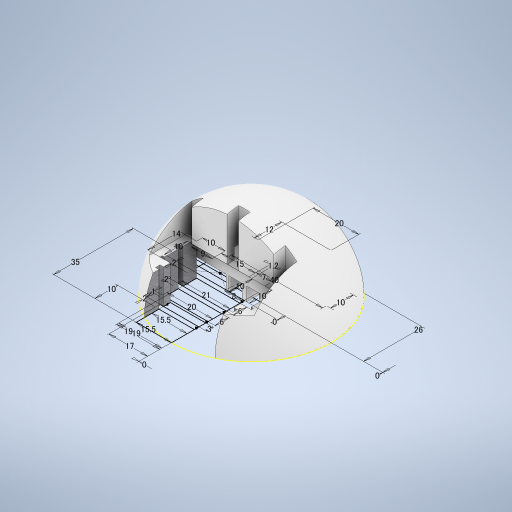
# Autodesk Inventor part: body back for tire1
Saved by Autodesk Inventor 2023 (Build 270158000, 158)
## iProperties
Created: 2022-10-08
Part Number: body back for tire1
Material: ABS プラスチック
Document SubType Name: Modeling
Designer: ellie
Density: 1.06 g/cm^3
Appearance: 積雪
Author: ellie
Autodesk Inventor part; units mm, degrees
sketch "スケッチ1" plane through (0, 0, 0) normal (0, 1, 0) x (-1, 0, 0)
  circle A0 centre (0, 0) radius 35
  line L0 (0, 0) -> (0, -35)
  line L1 (0, 0) -> (0, 35)
  dimension "d0" = 70
  constraints: 4 end point, 2 point on circle, 2 vertical, 1 centre point, 1 coincident
  measures "d0" diameter of A0
revolve "回転1" add sketch "スケッチ1" angle 180 about axis through (0, 0, 0) along (0, 0, 1) picked at (-2.5961, -23.0408) contours L1 L0 A0
sketch "スケッチ5" plane through (0, 0, 0) normal (0, -1, 0) x (1, 0, 0)
  line L0 (-20, -23) -> (20, -23)
  line L1 (20, -23) -> (20, -13)
  line L2 (20, -13) -> (-20, -13)
  line L3 (-20, -13) -> (-20, -23)
  line L4 (-20, -15) -> (-20, -13)
  line L5 (0, 25) -> (-17, 25)
  line L6 (-17, 25) -> (-17, 23)
  line L7 (-17, 23) -> (0, 23)
  line L8 (0, 23) -> (0, 25)
  line L9 (0, 20) -> (-20, 20)
  line L10 (-20, 20) -> (-20, 19)
  line L11 (-20, 19) -> (0, 19)
  line L12 (0, 19) -> (0, 20)
  line L13 (0, 13) -> (-21, 13)
  line L14 (-21, 13) -> (-21, 11)
  line L15 (-21, 11) -> (0, 11)
  line L16 (0, 11) -> (0, 13)
  line L17 (0, 5) -> (-23, 5)
  line L18 (-23, 5) -> (-23, 3)
  line L19 (-23, 3) -> (0, 3)
  line L20 (0, 3) -> (0, 5)
  circle A0 centre (0, 0) radius 35 projected
  circle A1 centre (0, 0) radius 35 projected
  line L21 (0, 35) -> (0, -35)
  line L22 (35, 0) -> (-35, 0)
  line L23 (-32, 3) -> (-23, 3)
  line L24 (-23, 3) -> (-23, -7)
  line L25 (-23, -7) -> (-32, -7)
  line L26 (-32, -7) -> (-32, 3)
  line L27 (-23, -8.0262) -> (-23, 3)
  line L28 (-15.5, 25) -> (0, 25)
  line L29 (0, 25) -> (0, 35)
  line L30 (0, 35) -> (-15.5, 35)
  line L31 (-15.5, 35) -> (-15.5, 25)
  line L32 (-15.5, 23) -> (0, 23)
  line L33 (0, 23) -> (0, 20)
  line L34 (0, 20) -> (-15.5, 20)
  line L35 (-15.5, 20) -> (-15.5, 23)
  line L36 (-19, 13) -> (0, 13)
  line L37 (0, 13) -> (0, 19)
  line L38 (0, 19) -> (-19, 19)
  line L39 (-19, 19) -> (-19, 13)
  line L40 (-19, 11) -> (0, 11)
  line L41 (0, 11) -> (0, 5)
  line L42 (0, 5) -> (-19, 5)
  line L43 (-19, 5) -> (-19, 11)
  line L44 (-23, -2) -> (-39.6865, -2)
  line L45 (-23, -2) -> (-7.8337, -2)
  line L46 (-8, 3) -> (-23, 3)
  line L47 (-23, 3) -> (-23, -7)
  line L48 (-23, -7) -> (-8, -7)
  line L49 (-8, -7) -> (-8, 3)
  line L50 (-8, 3) -> (-23, -7) construction
  line L51 (-23, 3) -> (-8, -7) construction
  line L52 (-23, 5) -> (-33, 5)
  line L53 (-33, 5) -> (-33, -9)
  line L54 (-33, -9) -> (-23, -9)
  line L55 (-23, -9) -> (-23, 5)
  line L56 (-23, 5) -> (-33, -9) construction
  line L57 (-33, 5) -> (-23, -9) construction
  line L58 (-8, 3) -> (-1, 3)
  line L59 (-1, 3) -> (-1, -7)
  line L60 (-1, -7) -> (-8, -7)
  line L61 (-8, -7) -> (-8, 3)
  line L62 (-8, 3) -> (-1, -7) construction
  line L63 (-1, 3) -> (-8, -7) construction
  line L64 (-23, 3) -> (-27, 3)
  line L65 (-23, -7) -> (-27, -7)
  line L66 (-23, 5) -> (-27, 5)
  line L67 (-23, -9) -> (-27, -9)
  line L68 (23.4307, -26) -> (-23.4307, -26)
  line L69 (-8, 3) -> (-6.8, 3)
  line L70 (-6.8, 3) -> (-6.8, -7)
  line L71 (-6.8, -7) -> (-8, -7)
  line L72 (-8, -7) -> (-8, 3)
  line L73 (-3, 5) -> (0, 5)
  line L74 (0, 20) -> (-4, 20)
  line L75 (-4, 19) -> (0, 19)
  line L76 (0, 19) -> (0, 20)
  line L77 (-6, 5) -> (-1, 5)
  line L78 (-1, 3) -> (-6, 3)
  line L79 (-33, -11.6619) -> (-33, 11.6619)
  point P0 (0, -23)
  point P1 (0, -13)
  point P2 (0, 24)
  point P3 (0, 19.5)
  point P4 (0, 12)
  point P5 (0, 4)
  point P6 (-20, -18)
  point P7 (-15.5, 21.5)
  point P8 (-15.5, 31.3807)
  point P9 (0, 25)
  point P10 (0, 23)
  point P11 (0, 11)
  point P12 (0, 13)
  point P13 (-32, 0)
  point P14 (-23, 0)
  point P15 (-15.5, -2)
  point P16 (-28, -2)
  point P17 (-4.5, -2)
  point P18 (-8, 3)
  point P19 (-28, 0.4738)
  point P20 (-28, -11.5262)
  point P21 (-23, -7)
  point P22 (-23, -7)
  point P23 (-23, -7)
  point P24 (-8, 0)
  point P25 (-1, 0)
  point P26 (0, 19)
  point P27 (0, 20)
  point P28 (-34.9428, -2)
  point P29 (-33, 11.6619)
  dimension "d12" = 40
  dimension "d13" = 10
  dimension "d23" = 17
  dimension "d24" = 2
  dimension "d27" = 20
  dimension "d28" = 1
  dimension "d30" = 21
  dimension "d31" = 2
  dimension "d33" = 2
  dimension "d88" = 0
  dimension "d89" = 0
  dimension "d90" = 12
  dimension "d92" = 20
  dimension "d93" = 10
  dimension "d97" = 9
  dimension "d98" = 10
  dimension "d122" = 15.5
  dimension "d123" = 35
  dimension "d124" = 3
  dimension "d125" = 15.5
  dimension "d126" = 6
  dimension "d127" = 6
  dimension "d128" = 19
  dimension "d129" = 19
  dimension "d147" = 10
  dimension "d149" = 8
  dimension "d151" = 15
  dimension "d161" = 14
  dimension "d162" = 10
  dimension "d164" = 10
  dimension "d165" = 7
  dimension "d170" = 26
  dimension "d175" = 1.2
  dimension "d207" = 0
  constraints: 158 end point, 31 parallel, 20 horizontal, 15 midpoint, 15 point on line, 14 perpendicular, 10 collinear, 21 other
  measures "d12" distance of L2.end L1.end
  measures "d13" distance of L1.end L0.end
  measures "d23" distance of L7.end L6.end
  measures "d24" distance of L6.end L5.end
  measures "d27" distance of L11.end L10.end
  measures "d28" distance of L10.end L9.end
  measures "d30" distance of L15.end L14.end
  measures "d31" distance of L14.end L13.end
  measures "d33" distance of L18.end L17.end
  measures "d89" distance from line of point (0, 0) L22
  measures "d90" distance from line of L0 point (0, -35)
  measures "d92" distance of the line from the sketch origin of L3
  measures "d93" distance from line of L5 point (0, 35)
  measures "d97" distance of L24.end L25.end
  measures "d98" distance of L23.end L24.end
  measures "d122" distance of the line from the sketch origin of L31
  measures "d123" distance between parallel lines of L30 L22
  measures "d124" distance of L32.end L33.end
  measures "d126" distance of L37.end L36.end
  measures "d127" distance of L40.end L41.end
  measures "d128" distance of the line from the sketch origin of L43
  measures "d129" distance of the line from the sketch origin of L39
  measures "d147" distance of L47.end L46.end
  measures "d149" distance of the line from the sketch origin of L49
  measures "d151" distance between parallel lines of L49 L24
  measures "d161" distance between parallel lines of L54 L52
  measures "d162" distance between parallel lines of L47 L53
  measures "d164" distance between parallel lines of L60 L58
  measures "d165" distance between parallel lines of L49 L59
  measures "d170" distance between parallel lines of L68 L22
  measures "d175" distance of L70.end L71.end
  measures "d207" distance between parallel lines of L46 L19
extrude "GNSボード" cut sketch "スケッチ5" against normal blind 16 contours L8 L7 L6 L5
extrude "GNSボード止めるよう" cut sketch "スケッチ5" against normal blind 15 contours L21 L5 L31 A0 | L21 L9 L35 L7
extrude "アルミ板１" cut sketch "スケッチ5" against normal blind 20 contours L11 L10 L9 L12
extrude "メイン基板" cut sketch "スケッチ5" against normal blind 21 contours L15 L14 L13 L16
extrude "メイン止めるよう" cut sketch "スケッチ5" against normal blind 15 contours L17 L43 L15 L21 | L13 L39 L11 L21
extrude "アルミ板２" cut sketch "スケッチ5" against normal blind 20 contours L19 L18 L17 L20
extrude "電池ボックス入れ" cut sketch "スケッチ5" against normal blind 13 contours L3 L2 L21 L0 | L21 L2 L1 L0
extrude "motor case" add sketch "スケッチ5" against normal blind 7 contours L53 L44 L26 L25 L27 L55 L54 | L49 L45 L24 L22 | L22 L24 L19 L49 | L53 L22 L26 L44 | L24 L44 L26 L22 | L22 L26 L23 L24 | L49 L48 L24 L45 | L53 L52 L18 L23 L26 L22 | L44 L24 L25 L26
extrude "bottom cut" cut sketch "スケッチ5" against normal blind 90 contours L68 A0 L21 | L21 A0 L68
extrude "motor" cut sketch "スケッチ5" against normal blind 6 contours L59 L60 L70 L22 | L22 L70 L19 L59 | L70 L60 L49 L22 | L22 L49 L19 L70 | L49 L45 L24 L22 | L22 L24 L19 L49 | L24 L44 L26 L22 | L22 L26 L23 L24 | L49 L48 L24 L45 | L44 L24 L25 L26
extrude "motor block" add sketch "スケッチ5" against normal blind 10 contours L70 L60 L49 L22 | L22 L49 L19 L70
mirror "ミラー13" about plane through (0, 0, 0) normal (1, 0, 0) of "メイン止めるよう", "メイン基板", "アルミ板１", "GNSボード止めるよう", "GNSボード", "アルミ板２", "motor", "motor case", "電池ボックス入れ", "motor block"
ref_plane "作業平面5" through (-17, 17.5, 23) normal (0, -1, 0) x (1, 0, 0)
ref_plane "作業平面6" through (20, 13, -13) normal (0, 0, -1) x (1, 0, 0)
ref_plane "作業平面7" through (27, 35, 5) normal (0, -1, 0) x (1, 0, 0)
sketch "スケッチ41" plane through (-17, 0, 23) normal (0, -1, 0) x (1, 0, 0)
  line L0 (-15, -30) -> (-15, -20) projected
  line L1 (-15, -20) -> (-6, -20) projected
  line L2 (-6, -20) -> (-6, -18) projected
  line L3 (-6, -18) -> (-2, -18) projected
  line L4 (-2, -18) -> (-2, -12) projected
  line L5 (-2, -12) -> (-4, -12) projected
  line L6 (-4, -12) -> (-4, -10) projected
  line L7 (-4, -10) -> (-2, -10) projected
  line L8 (-2, -10) -> (-2, -4) projected
  line L9 (-2, -4) -> (-3, -4) projected
  line L10 (-3, -4) -> (-3, -3) projected
  line L11 (-3, -3) -> (1.5, -3) projected
  line L12 (1.5, -3) -> (1.5, 0) projected
  line L13 (1.5, 0) -> (0, 0) projected
  line L14 (0, 0) -> (0, 2) projected
  line L15 (0, 2) -> (1.5, 2) projected
  line L16 (1.5, 2) -> (1.5, 8.3807) projected
  arc A0 (1.5, 8.3807) -> (-6.4307, -49) centre (17, -23) ccw projected
  line L17 (-2, -18) -> (-2, -12) projected
  line L18 (-4, -10) -> (-4, -12) projected
  line L19 (0, 2) -> (0, 0) projected
  circle A1 centre (-4, 0.5) radius 2.4
  line L20 (18, -30) -> (18, -20) projected
  line L21 (18, -20) -> (16, -20) projected
  line L22 (16, -20) -> (16, -30) projected
  line L23 (16, -30) -> (10.2, -30) projected
  line L24 (10.2, -30) -> (10.2, -20) projected
  line L25 (10.2, -20) -> (9, -20) projected
  line L26 (9, -20) -> (9, -30) projected
  line L27 (9, -30) -> (-15, -30) projected
  line L28 (-6.4307, -49) -> (40.4307, -49) projected
  arc A2 (40.4307, -49) -> (32.5, 8.3807) centre (17, -23) ccw projected
  line L29 (32.5, 8.3807) -> (32.5, 2) projected
  line L30 (32.5, 2) -> (34, 2) projected
  line L31 (34, 2) -> (34, 0) projected
  line L32 (34, 0) -> (32.5, 0) projected
  line L33 (32.5, 0) -> (32.5, -3) projected
  line L34 (32.5, -3) -> (37, -3) projected
  line L35 (37, -3) -> (37, -4) projected
  line L36 (37, -4) -> (36, -4) projected
  line L37 (36, -4) -> (36, -10) projected
  line L38 (36, -10) -> (38, -10) projected
  line L39 (38, -10) -> (38, -12) projected
  line L40 (38, -12) -> (36, -12) projected
  line L41 (36, -12) -> (36, -18) projected
  line L42 (36, -18) -> (40, -18) projected
  line L43 (40, -18) -> (40, -20) projected
  line L44 (40, -20) -> (49, -20) projected
  line L45 (49, -20) -> (49, -30) projected
  line L46 (49, -30) -> (25, -30) projected
  line L47 (25, -20) -> (25, -30) projected
  line L48 (23.8, -20) -> (25, -20) projected
  line L49 (23.8, -30) -> (23.8, -20) projected
  line L50 (23.8, -30) -> (18, -30) projected
  dimension "d252" = 4.8
  dimension "d253" = 4
  dimension "d254" = 3.5
  constraints: 1 centre point
  measures "d252" diameter of A1
  measures "d253" distance from line of A1.centre L14
  measures "d254" distance from line of A1.centre L11
extrude "top lock 10mm" cut sketch "スケッチ41" against normal blind 3 contours A1
mirror "ミラー15" about plane through (0, 0, 0) normal (1, 0, 0) of "top lock 10mm"
ref_plane "作業平面9" through (-33, 0, -9) normal (0, -1, 0) x (1, 0, 0)
sketch "スケッチ42" plane through (-33, 0, -9) normal (0, -1, 0) x (1, 0, 0)
  circle A0 centre (9.5, -3) radius 2.4
  line L0 (13, -14) -> (13, -4) projected
  line L1 (32, 2) -> (1, 2) projected
  point P0 (33, 9)
  point P1 (10, 2)
  dimension "d257" = 3.5
  dimension "d258" = 4.8
  dimension "d259" = 5
  constraints: 1 centre point
  measures "d257" distance from line of A0.centre L0
  measures "d258" diameter of A0
  measures "d259" distance from line of A0.centre L1
extrude "bottom lock" cut sketch "スケッチ42" against normal blind 3
ref_plane "作業平面8" through (-17, 15, 23) normal (0, -1, 0) x (1, 0, 0)
sketch "スケッチ45" plane through (-17, 15, 23) normal (0, -1, 0) x (1, 0, 0)
  circle A0 centre (-4, 0.5) radius 2.4 projected
  line L0 (-15, -30) -> (-15, -20) projected
  line L1 (-15, -20) -> (-6, -20) projected
  line L2 (-6, -20) -> (-6, -18) projected
  line L3 (-6, -18) -> (-2, -18) projected
  line L4 (-2, -18) -> (-2, -12) projected
  line L5 (-2, -12) -> (-4, -12) projected
  line L6 (-4, -12) -> (-4, -10) projected
  line L7 (-4, -10) -> (-2, -10) projected
  line L8 (-2, -10) -> (-2, -4) projected
  line L9 (-2, -4) -> (-3, -4) projected
  line L10 (-3, -4) -> (-3, -3) projected
  line L11 (-3, -3) -> (1.5, -3) projected
  line L12 (1.5, -3) -> (1.5, 0) projected
  line L13 (1.5, 0) -> (0, 0) projected
  line L14 (0, 0) -> (0, 2) projected
  line L15 (0, 2) -> (1.5, 2) projected
  line L16 (1.5, 2) -> (1.5, 8.3807) projected
  arc A1 (1.5, 8.3807) -> (-6.4307, -49) centre (17, -23) ccw projected
  arc A2 (32.5, 4.5636) -> (1.5, 4.5636) centre (17, -23) ccw projected
  line L17 (1.5, 2) -> (1.5, 4.5636) projected
  line L18 (32.5, 2) -> (1.5, 2) projected
  line L19 (32.5, 2) -> (32.5, 4.5636) projected
  circle A3 centre (38, 0.5) radius 2.4 projected
  arc A4 (40.4307, -49) -> (32.5, 8.3807) centre (17, -23) ccw projected
  line L20 (32.5, 8.3807) -> (32.5, 2) projected
  line L21 (32.5, 2) -> (34, 2) projected
  line L22 (34, 2) -> (34, 0) projected
  line L23 (34, 0) -> (32.5, 0) projected
  line L24 (32.5, 0) -> (32.5, -3) projected
  line L25 (32.5, -3) -> (37, -3) projected
  line L26 (37, -3) -> (37, -4) projected
  line L27 (37, -4) -> (36, -4) projected
  line L28 (36, -4) -> (36, -10) projected
  line L29 (36, -10) -> (38, -10) projected
  line L30 (38, -10) -> (38, -12) projected
  line L31 (38, -12) -> (36, -12) projected
  line L32 (36, -12) -> (36, -18) projected
  line L33 (36, -18) -> (40, -18) projected
  line L34 (40, -18) -> (40, -20) projected
  line L35 (40, -20) -> (49, -20) projected
  line L36 (49, -20) -> (49, -30) projected
  circle A5 centre (38, 0.5) radius 2.4 projected
  circle A6 centre (-4, 0.5) radius 2.4 projected
  line L37 (34, 0) -> (0, 0) projected
  line L38 (34, 0) -> (34, 2) projected
  line L39 (34, 2) -> (0, 2) projected
  line L40 (0, 0) -> (0, 2) projected
  line L41 (32.5, -3) -> (1.5, -3) projected
  line L42 (32.5, -3) -> (32.5, 0) projected
  line L43 (1.5, 0) -> (32.5, 0) projected
  line L44 (1.5, -3) -> (1.5, 0) projected
  line L45 (-2, -4) -> (36, -4) projected
  circle A7 centre (38, 0.5) radius 2.4 projected
  line L46 (36, -10) -> (-2, -10) projected
  line L47 (36, -10) -> (36, -4) projected
  line L48 (-2, -4) -> (36, -4) projected
  line L49 (-2, -10) -> (-2, -4) projected
  line L50 (-2, -12) -> (36, -12) projected
  line L51 (36, -18) -> (-2, -18) projected
  line L52 (36, -18) -> (36, -12) projected
  line L53 (-2, -12) -> (36, -12) projected
  line L54 (-2, -18) -> (-2, -12) projected
  line L55 (40, -20) -> (-6, -20) projected
  line L56 (40, -20) -> (40, -18) projected
  line L57 (40, -18) -> (-6, -18) projected
  line L58 (-6, -20) -> (-6, -18) projected
  line L59 (9, -30) -> (9, -20) projected
  line L60 (-6, -20) -> (9, -20) projected
  line L61 (-15, -20) -> (-6, -20) projected
  line L62 (-15, -30) -> (-15, -20) projected
  line L63 (16, -30) -> (10.2, -30) projected
  line L64 (18, -30) -> (18, -20) projected
  line L65 (18, -20) -> (16, -20) projected
  line L66 (16, -20) -> (16, -30) projected
  line L67 (-6, -20) -> (-6, -18) projected
  line L68 (16, -30) -> (10.2, -30) projected
  line L69 (-15, -30) -> (-15, -20) projected
  arc A8 (1.5, 8.3807) -> (-6.4307, -49) centre (17, -23) ccw projected
  line L70 (-6.4307, -49) -> (40.4307, -49) projected
  arc A9 (40.4307, -49) -> (32.5, 8.3807) centre (17, -23) ccw projected
  line L71 (49, -20) -> (49, -30) projected
  line L72 (23.8, -30) -> (18, -30) projected
  line L73 (40, -18) -> (40, -20) projected
  line L74 (-3, -36) -> (37, -36) projected
  line L75 (37, -36) -> (37, -46) projected
  line L76 (37, -46) -> (-3, -46) projected
  line L77 (-3, -46) -> (-3, -36) projected
  line L78 (-6, -15) -> (40, -15)
  line L79 (40, -15) -> (40, 8.6228)
  line L80 (40, 8.6228) -> (-6, 8.6228)
  line L81 (-6, 8.6228) -> (-6, -15)
  line L82 (10.2, -20) -> (10.2, -30) projected
  line L83 (16, -20) -> (16, -30) projected
  line L84 (10.2, -20) -> (16, -20) projected
  line L85 (9, -30) -> (-15, -30) projected
  line L86 (-15, -20) -> (-6, -20) projected
  line L87 (-6, -18) -> (-2, -18) projected
  line L88 (-2, -18) -> (-2, -12) projected
  line L89 (-2, -12) -> (-4, -12) projected
  line L90 (-4, -12) -> (-4, -10) projected
  line L91 (-4, -10) -> (-2, -10) projected
  line L92 (-2, -10) -> (-2, -4) projected
  line L93 (-2, -4) -> (-3, -4) projected
  line L94 (-3, -4) -> (-3, -3) projected
  line L95 (-3, -3) -> (1.5, -3) projected
  line L96 (1.5, -3) -> (1.5, 0) projected
  line L97 (1.5, 0) -> (0, 0) projected
  line L98 (0, 0) -> (0, 2) projected
  line L99 (0, 2) -> (1.5, 2) projected
  line L100 (1.5, 2) -> (1.5, 8.3807) projected
  line L101 (10.2, -30) -> (10.2, -20) projected
  line L102 (10.2, -20) -> (9, -20) projected
  line L103 (9, -20) -> (9, -30) projected
  line L104 (9, -30) -> (-15, -30) projected
  line L105 (49, -30) -> (25, -30) projected
  line L106 (25, -20) -> (25, -30) projected
  line L107 (23.8, -20) -> (25, -20) projected
  line L108 (23.8, -30) -> (23.8, -20) projected
  line L109 (32.5, 8.3807) -> (32.5, 2) projected
  line L110 (32.5, 2) -> (34, 2) projected
  line L111 (34, 2) -> (34, 0) projected
  line L112 (34, 0) -> (32.5, 0) projected
  line L113 (32.5, 0) -> (32.5, -3) projected
  line L114 (32.5, -3) -> (37, -3) projected
  line L115 (37, -3) -> (37, -4) projected
  line L116 (37, -4) -> (36, -4) projected
  line L117 (36, -4) -> (36, -10) projected
  line L118 (36, -10) -> (38, -10) projected
  line L119 (38, -10) -> (38, -12) projected
  line L120 (38, -12) -> (36, -12) projected
  line L121 (36, -12) -> (36, -18) projected
  line L122 (36, -18) -> (40, -18) projected
  line L123 (40, -20) -> (49, -20) projected
  line L124 (18, -30) -> (18, -20) projected
  line L125 (18, -20) -> (16, -20) projected
  line L126 (16, -20) -> (16, -30) projected
  line L127 (16, -30) -> (10.2, -30) projected
  line L128 (10.2, -30) -> (10.2, -20) projected
  line L129 (10.2, -20) -> (9, -20) projected
  line L130 (9, -20) -> (9, -30) projected
  line L131 (9, -30) -> (-15, -30) projected
  line L132 (-15, -30) -> (-15, -20) projected
  line L133 (-15, -20) -> (-6, -20) projected
  line L134 (-6, -20) -> (-6, -18) projected
  line L135 (-6, -18) -> (-2, -18) projected
  line L136 (-2, -18) -> (-2, -12) projected
  line L137 (-2, -12) -> (-4, -12) projected
  line L138 (-4, -12) -> (-4, -10) projected
  line L139 (-4, -10) -> (-2, -10) projected
  line L140 (-2, -10) -> (-2, -4) projected
  line L141 (-2, -4) -> (-3, -4) projected
  line L142 (-3, -4) -> (-3, -3) projected
  line L143 (-3, -3) -> (1.5, -3) projected
  line L144 (1.5, -3) -> (1.5, 0) projected
  line L145 (1.5, 0) -> (0, 0) projected
  line L146 (0, 0) -> (0, 2) projected
  line L147 (0, 2) -> (1.5, 2) projected
  line L148 (1.5, 2) -> (1.5, 8.3807) projected
  arc A10 (1.5, 8.3807) -> (-6.4307, -49) centre (17, -23) ccw projected
  line L149 (-6.4307, -49) -> (40.4307, -49) projected
  line L150 (49, -30) -> (25, -30) projected
  line L151 (25, -20) -> (25, -30) projected
  line L152 (23.8, -20) -> (25, -20) projected
  line L153 (23.8, -30) -> (23.8, -20) projected
  line L154 (23.8, -30) -> (18, -30) projected
  line L155 (18, -30) -> (18, -20) projected
  line L156 (18, -20) -> (16, -20) projected
  line L157 (16, -20) -> (16, -30) projected
  line L158 (16, -30) -> (10.2, -30) projected
  line L159 (10.2, -30) -> (10.2, -20) projected
  line L160 (10.2, -20) -> (9, -20) projected
  line L161 (9, -20) -> (9, -30) projected
  line L162 (9, -30) -> (-15, -30) projected
  line L163 (-6.4307, -49) -> (40.4307, -49) projected
  arc A11 (40.4307, -49) -> (32.5, 8.3807) centre (17, -23) ccw projected
  line L164 (32.5, 8.3807) -> (32.5, 2) projected
  line L165 (32.5, 2) -> (34, 2) projected
  line L166 (34, 2) -> (34, 0) projected
  line L167 (34, 0) -> (32.5, 0) projected
  line L168 (32.5, 0) -> (32.5, -3) projected
  line L169 (32.5, -3) -> (37, -3) projected
  line L170 (37, -3) -> (37, -4) projected
  line L171 (37, -4) -> (36, -4) projected
  line L172 (36, -4) -> (36, -10) projected
  line L173 (36, -10) -> (38, -10) projected
  line L174 (38, -10) -> (38, -12) projected
  line L175 (38, -12) -> (36, -12) projected
  line L176 (36, -12) -> (36, -18) projected
  line L177 (36, -18) -> (40, -18) projected
  line L178 (40, -18) -> (40, -20) projected
  line L179 (40, -20) -> (49, -20) projected
  line L180 (49, -20) -> (49, -30) projected
  line L181 (49, -30) -> (25, -30) projected
  line L182 (25, -20) -> (25, -30) projected
  line L183 (23.8, -20) -> (25, -20) projected
  line L184 (23.8, -30) -> (23.8, -20) projected
  line L185 (23.8, -30) -> (18, -30) projected
  dimension "d269" = 3
  constraints: 8 end point, 2 collinear, 2 parallel, 1 horizontal, 1 perpendicular, 1 tangent
  measures "d269" distance between parallel lines of L78 L57
extrude "back cut" cut sketch "スケッチ45" against normal blind 20 contours A0 L81 | A0 L81 A1 L16 L15 L14 L13 L12 L11 L10 L9 L8 L7 L6 L5 L4 L78 | L81 L80 A2 L16 A1 | L4 L50 L32 L78 | A2 L19 L18 L16 | L80 L79 A4 L20 A2 | L5 L6 L7 L46 L29 L30 L31 L50 | L32 L31 L30 L29 L28 L27 L26 L25 L24 L23 L22 L21 L19 L20 A4 L79 A3 L78 | L18 L21 L22 L23 L37 L13 L14 L15 | L79 A3 | L8 L45 L28 L46 | L37 L24 L41 L12 | L9 L10 L11 L41 L25 L26 L27 L45 picked at (-4.4805, 1.0136) picked at (36.1523, 0.5971)
sketch "スケッチ52" plane through (20, 0, -13) normal (0, 0, -1) x (-1, 0, 0)
  line L0 (40, 0) -> (0, 0) projected
  line L1 (40, 0) -> (40, 13) projected
  line L2 (40, 13) -> (0, 13) projected
  line L3 (0, 0) -> (0, 13) projected
  line L4 (28, 0) -> (28, 6) projected
  line L5 (28, 6) -> (52, 6) projected
  line L6 (52, 0) -> (52, 6) projected
  line L7 (28, 0) -> (52, 0) projected
  line L8 (26.8, 6) -> (26.8, 0) projected
  line L9 (21, 0) -> (26.8, 0) projected
  line L10 (21, 0) -> (21, 6) projected
  line L11 (21, 6) -> (26.8, 6) projected
  line L12 (13.2, 0) -> (13.2, 6) projected
  line L13 (19, 6) -> (13.2, 6) projected
  line L14 (19, 0) -> (19, 6) projected
  line L15 (13.2, 0) -> (19, 0) projected
  line L16 (12, 6) -> (12, 0) projected
  line L17 (-12, 0) -> (12, 0) projected
  line L18 (-12, 0) -> (-12, 6) projected
  line L19 (12, 6) -> (-12, 6) projected
  line L20 (27, 10) -> (37, 10)
  line L21 (37, 10) -> (37, 16)
  line L22 (37, 16) -> (27, 16)
  line L23 (27, 16) -> (27, 10)
  point P0 (20, 0)
  dimension "d293" = 3
  dimension "d294" = 10
  dimension "d295" = 4
  constraints: 8 end point, 2 parallel, 1 horizontal, 1 perpendicular, 1 other
  measures "d293" distance between parallel lines of L1 L21
  measures "d294" distance between parallel lines of L21 L23
  measures "d295" distance between parallel lines of L20 L5
extrude "押し出し54" cut sketch "スケッチ52" against normal up to surface (18 mm away) contours L21 L20 L23 L2 | L2 L23 L22 L21
sketch "スケッチ53" plane through (0, 13, 0) normal (0, -1, 0) x (1, 0, 0)
  line L0 (-7, -13) -> (-7, 3) projected
  line L1 (-17, -13) -> (-7, -13) projected
  line L2 (-17, -13) -> (-17, 3) projected
  line L3 (-17, -13) -> (-17, 3) projected
  line L4 (-17, -13) -> (-17, 3) projected
  line L5 (-23, 8) -> (23, 8) projected
  line L6 (23, 8) -> (23, 21.7025) projected
  arc A0 (23, 21.7025) -> (15.5, 27.5636) centre (0, 0) ccw projected
  line L7 (15.5, 27.5636) -> (15.5, 31.3807) projected
  arc A1 (23.4307, -26) -> (15.5, 31.3807) centre (0, 0) ccw projected
  line L8 (23.4307, -26) -> (-23.4307, -26) projected
  arc A2 (-15.5, 31.3807) -> (-23.4307, -26) centre (0, 0) ccw projected
  line L9 (-15.5, 31.3807) -> (-15.5, 27.5636) projected
  arc A3 (-15.5, 27.5636) -> (-23, 21.7025) centre (0, 0) ccw projected
  line L10 (-23, 21.7025) -> (-23, 8) projected
  line L11 (-17, -13) -> (-7, -13)
  line L12 (-7, -13) -> (-7, -19)
  line L13 (-7, -19) -> (-17, -19)
  line L14 (-17, -19) -> (-17, -13)
  dimension "d298" = 6
  constraints: 8 end point, 3 collinear, 2 parallel, 1 horizontal, 1 perpendicular
  measures "d298" distance between parallel lines of L13 L1
extrude "押し出し55" cut sketch "スケッチ53" against normal up to surface (3 mm away) contours L1 L12 L13 L14
sketch "スケッチ54" plane through (-23, 15, 8) normal (0, 0, 1) x (1, 0, 0)
  line L0 (42, 0) -> (46, 0) projected
  line L1 (46, 0) -> (41, 0)
  line L2 (41, 0) -> (41, 20)
  line L3 (41, 20) -> (46, 20)
  line L4 (46, 20) -> (46, 0)
  line L5 (0, 0) -> (4, 0) projected
  line L6 (0, 0) -> (5, 0)
  line L7 (5, 0) -> (5, 20)
  line L8 (5, 20) -> (0, 20)
  line L9 (0, 20) -> (0, 0)
  line L10 (23, -15) -> (23, 20)
  arc A0 (58, -15) -> (-12, -15) centre (23, -15) ccw projected
  line L11 (25.5, 0) -> (20.5, 0)
  line L12 (20.5, 0) -> (20.5, 20)
  line L13 (20.5, 20) -> (25.5, 20)
  line L14 (25.5, 20) -> (25.5, 0)
  line L15 (42, 0) -> (4, 0) projected
  arc A1 (46, 10.1396) -> (0, 10.1396) centre (23, -15) ccw projected
  line L16 (0, 0) -> (0, 10.1396) projected
  line L17 (0, 0) -> (4, 0) projected
  line L18 (42, 0) -> (4, 0) projected
  line L19 (42, 0) -> (46, 0) projected
  line L20 (46, 0) -> (46, 10.1396) projected
  line L21 (46, 0) -> (38.5, 0) projected
  line L22 (38.5, 0) -> (38.5, -15) projected
  line L23 (38.5, -15) -> (46.4307, -15) projected
  arc A2 (46.4307, -15) -> (-0.4307, -15) centre (23, -15) ccw projected
  line L24 (-0.4307, -15) -> (7.5, -15) projected
  line L25 (7.5, -15) -> (7.5, 0) projected
  line L26 (7.5, 0) -> (0, 0) projected
  line L27 (0, 0) -> (0, 10.1396) projected
  arc A3 (46, 10.1396) -> (0, 10.1396) centre (23, -15) ccw projected
  line L28 (46, 10.1396) -> (46, 0) projected
  point P0 (20.5, 0)
  point P1 (20.5, 19.9106)
  point P2 (5, 15.0167)
  point P3 (41, 15.0167)
  point P4 (25.5, 19.9106)
  point P5 (25.5, 0)
  point P6 (41, 13.931)
  point P7 (25.5, 18.9816)
  point P8 (20.5, 18.9816)
  point P9 (5, 13.931)
  point P10 (0, 10.1396)
  point P11 (46, 11.3818)
  point P12 (0, 11.3818)
  dimension "d301" = 5
  dimension "d302" = 5
  dimension "d303" = 2.5
  dimension "d304" = 5
  constraints: 26 end point, 6 parallel, 3 horizontal, 3 perpendicular, 3 tangent, 1 collinear, 1 point on circle, 1 vertical
  measures "d301" distance of L2.end L3.end
  measures "d302" distance of L8.end L7.end
  measures "d303" distance between parallel lines of L14 L10
  measures "d304" distance between parallel lines of L14 L12
extrude "押し出し56" cut sketch "スケッチ54" against normal up to surface (5 mm away) contours L1 L2 A1 L4 L0 | A1 L2 A0 L4 | A2 L10 A1 L14 | L14 L11 L10 A2 | A1 L10 A0 L14 | A2 L12 A1 L10 | L10 L11 L12 A2 | A0 L13 L14 | A1 L12 A0 L10 | A0 L12 L13 | L6 L5 L9 A1 L7 | A1 L9 A0 L7
extrude "押し出し60" cut sketch "スケッチ5" against normal blind 27 contours A0 L44 L53 L79 | A0 L22 L53 L44 | A0 L79 L53 L22
sketch "スケッチ60" plane through (-33, 0, -11.6619) normal (-1, 0, 0) x (0, 0, 1)
  line L0 (4.6619, 0) -> (14.6619, 0) projected
  circle A0 centre (9.6619, 0) radius 15
  point P0 (11.6619, 0)
  dimension "d320" = 30
  constraints: 1 centre point, 1 coincident, 1 midpoint
  measures "d320" diameter of A0
extrude "押し出し61" cut sketch "スケッチ60" against normal blind 6
sketch "スケッチ61" plane through (-23.4307, 0, -26) normal (0, -1, 0) x (1, 0, 0)
  line L0 (-9.0654, 39) -> (-3.5693, 39) projected
  line L1 (-3.5693, 39) -> (-3.5693, 29) projected
  line L2 (-3.5693, 19) -> (-3.5693, 9) projected
  line L3 (-3.5693, 9) -> (-7.1634, 9) projected
  line L4 (-3.5693, 9) -> (-3.5693, 39) projected
  line L5 (-9.0654, 39) -> (-3.5693, 39) projected
  point P0 (23.4307, 26)
  constraints: 1 other
